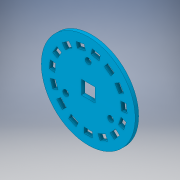
# Autodesk Inventor part: MountCover
Saved by Autodesk Inventor 2019.3 (Build 233278000, 278)
## iProperties
Created: 2018-12-24
Part Number: MountCover
Material: Polycarbonate, Clear
Document SubType Name: Modeling
Designer: steele
Density: 1.2 g/cm^3
Appearance: Sky Blue Medium
Author: steele
Comments: 1/11/19 Reduced the diamter of the outside by 2 mm so the part would fit better onto the main housing.
Autodesk Inventor part; units mm, degrees
ref_plane "YZ Plane" through (0, 0, 0) normal (1, 0, 0) x (0, 1, 0)
ref_plane "XZ Plane" through (0, 0, 0) normal (0, 1, 0) x (-1, 0, 0)
ref_plane "XY Plane" through (0, 0, 0) normal (0, 0, 1) x (1, 0, 0)
sketch "Sketch1" plane through (0, 0, 0) normal (0, 0, 1) x (1, 0, 0)
  circle A0 centre (0, 0) radius 34
  dimension "d0" = 68
  constraints: 1 centre point, 1 coincident
  measures "d0" diameter of A0
extrude "Extrusion1" add sketch "Sketch1" against normal blind 2.54
sketch "Sketch2" plane through (0, 0, -2.54) normal (0, 0, -1) x (-1, 0, 0)
  line L0 (5, 5) -> (-5, 5)
  line L1 (-5, 5) -> (-5, -5)
  line L2 (-5, -5) -> (5, -5)
  line L3 (5, -5) -> (5, 5)
  line L4 (5, 5) -> (-5, -5) construction
  line L5 (-5, 5) -> (5, -5) construction
  point P0 (0, 0)
  dimension "d3" = 10
  constraints: 12 end point, 2 midpoint, 2 parallel, 2 perpendicular, 1 horizontal
  measures "d3" distance of L1.end L2.end
extrude "Extrusion2" cut sketch "Sketch2" against normal through all
sketch "Sketch3" plane through (0, 0, -2.54) normal (0, 0, -1) x (-1, 0, 0)
  circle A0 centre (0, 0) radius 26 construction
  line L0 (3, -24) -> (-3, -24)
  line L1 (-3, -24) -> (-3, -28)
  line L2 (-3, -28) -> (3, -28)
  line L3 (3, -28) -> (3, -24)
  line L4 (3, -24) -> (-3, -28) construction
  line L5 (-3, -24) -> (3, -28) construction
  line L6 (8.648, -26.7995) -> (14.1293, -24.3591)
  line L7 (14.1293, -24.3591) -> (12.5023, -20.7049)
  line L8 (7.021, -23.1453) -> (8.648, -26.7995)
  line L9 (12.5023, -20.7049) -> (7.021, -23.1453)
  line L10 (18.8007, -20.9651) -> (22.8154, -16.5062)
  line L11 (22.8154, -16.5062) -> (19.8429, -13.8297)
  line L12 (15.8281, -18.2886) -> (18.8007, -20.9651)
  line L13 (19.8429, -13.8297) -> (15.8281, -18.2886)
  line L14 (25.7025, -11.5056) -> (27.5566, -5.7993)
  line L15 (27.5566, -5.7993) -> (23.7524, -4.5632)
  line L16 (21.8983, -10.2696) -> (25.7025, -11.5056)
  line L17 (23.7524, -4.5632) -> (21.8983, -10.2696)
  line L18 (28.1602, -0.0568) -> (27.533, 5.9104)
  line L19 (27.533, 5.9104) -> (23.5549, 5.4922)
  line L20 (24.1821, -0.4749) -> (28.1602, -0.0568)
  line L21 (23.5549, 5.4922) -> (24.1821, -0.4749)
  line L22 (25.7487, 11.4019) -> (22.7487, 16.5981)
  line L23 (22.7487, 16.5981) -> (19.2846, 14.5981)
  line L24 (22.2846, 9.4019) -> (25.7487, 11.4019)
  line L25 (19.2846, 14.5981) -> (22.2846, 9.4019)
  line L26 (18.885, 20.8891) -> (14.0309, 24.4158)
  line L27 (14.0309, 24.4158) -> (11.6798, 21.1798)
  line L28 (16.5339, 17.6531) -> (18.885, 20.8891)
  line L29 (11.6798, 21.1798) -> (16.5339, 17.6531)
  line L30 (8.756, 26.7644) -> (2.8871, 28.0119)
  line L31 (2.8871, 28.0119) -> (2.0554, 24.0993)
  line L32 (7.9243, 22.8518) -> (8.756, 26.7644)
  line L33 (2.0554, 24.0993) -> (7.9243, 22.8518)
  line L34 (-2.8871, 28.0119) -> (-8.756, 26.7644)
  line L35 (-8.756, 26.7644) -> (-7.9243, 22.8518)
  line L36 (-2.0554, 24.0993) -> (-2.8871, 28.0119)
  line L37 (-7.9243, 22.8518) -> (-2.0554, 24.0993)
  line L38 (-14.0309, 24.4158) -> (-18.885, 20.8891)
  line L39 (-18.885, 20.8891) -> (-16.5339, 17.6531)
  line L40 (-11.6798, 21.1798) -> (-14.0309, 24.4158)
  line L41 (-16.5339, 17.6531) -> (-11.6798, 21.1798)
  line L42 (-22.7487, 16.5981) -> (-25.7487, 11.4019)
  line L43 (-25.7487, 11.4019) -> (-22.2846, 9.4019)
  line L44 (-19.2846, 14.5981) -> (-22.7487, 16.5981)
  line L45 (-22.2846, 9.4019) -> (-19.2846, 14.5981)
  line L46 (-27.533, 5.9104) -> (-28.1602, -0.0568)
  line L47 (-28.1602, -0.0568) -> (-24.1821, -0.4749)
  line L48 (-23.5549, 5.4922) -> (-27.533, 5.9104)
  line L49 (-24.1821, -0.4749) -> (-23.5549, 5.4922)
  line L50 (-27.5566, -5.7993) -> (-25.7025, -11.5056)
  line L51 (-25.7025, -11.5056) -> (-21.8983, -10.2696)
  line L52 (-23.7524, -4.5632) -> (-27.5566, -5.7993)
  line L53 (-21.8983, -10.2696) -> (-23.7524, -4.5632)
  line L54 (-22.8154, -16.5062) -> (-18.8007, -20.9651)
  line L55 (-18.8007, -20.9651) -> (-15.8281, -18.2886)
  line L56 (-19.8429, -13.8297) -> (-22.8154, -16.5062)
  line L57 (-15.8281, -18.2886) -> (-19.8429, -13.8297)
  line L58 (-14.1293, -24.3591) -> (-8.648, -26.7995)
  line L59 (-8.648, -26.7995) -> (-7.021, -23.1453)
  line L60 (-12.5023, -20.7049) -> (-14.1293, -24.3591)
  line L61 (-7.021, -23.1453) -> (-12.5023, -20.7049)
  point P0 (0, -26)
  dimension "d6" = 52
  dimension "d7" = 4
  dimension "d8" = 6
  dimension "d11" = 360
  constraints: 124 end point, 2 midpoint, 2 parallel, 1 coincident, 1 horizontal, 1 perpendicular, 1 vertical alignment, 123 other
  measures "d7" distance of L2.end L0.start
  measures "d8" distance of L1.end L2.end
extrude "Extrusion3" cut sketch "Sketch3" against normal through all
sketch "Sketch4" plane through (0, 0, 0) normal (0, 0, 1) x (1, 0, 0)
  line L0 (-18.7521, 0) -> (0, 0) construction
  line L1 (0, 0) -> (0, 18.7521) construction
  circle A0 centre (0, 0) radius 18.7521 construction
  point P0 (-16.2398, -9.376)
  point P1 (16.2398, -9.3761)
  dimension "d15" = 37.5042
  dimension "d16" = 18.7521
  dimension "d17" = 90
  dimension "d20" = 360
  constraints: 4 end point, 2 coincident, 1 centre point, 1 horizontal, 1 perpendicular, 4 other
  measures "d15" diameter of A0
  measures "d16" distance of L0.end L1.end
  measures "d17" angle of L0 L1
hole "Hole1" at (0, 18.7521, 0) at (-16.2398, -9.376, 0) at (16.2398, -9.3761, 0) direction (0, 0, -1) diameter 4.318 end through all clearance for "Flat Head Machine Screw (82)" size "#6" standard "Ansi Unified Screw Threads"
equation "\"d1\" = CoverDepth"
equation "\"d6\" = 2 * LightRingCenterRadius"
equation "\"d15\" = SupportScrewsDiameter"
equation "\"d16\" = 0.5 * SupportScrewsDiameter"
equation "\"CoverDepth\" = 2.54"
equation "\"LightRingCenterRadius\" = 26"
equation "\"SupportScrewsDiameter\" = 37.5042"
body "Solid1"
